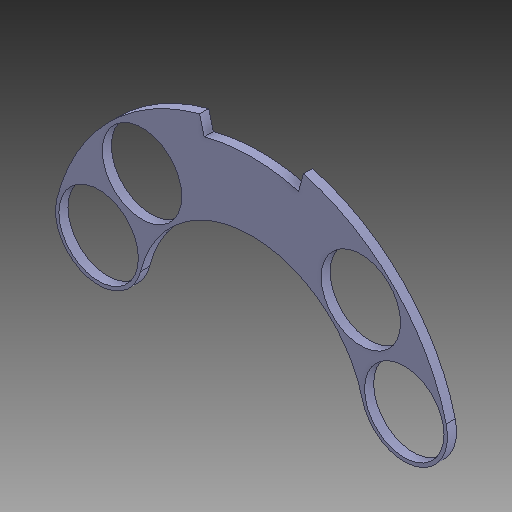
# Autodesk Inventor part: Диск_фиксатор
Saved by Autodesk Inventor 2022 (Build 260153000, 153)
## iProperties
Created: 2025-01-11
Part Number: Диск_фиксатор
Material: Типовые
Document SubType Name: Modeling
Designer: Ivan
Density: 1 g/cm^3
Appearance: Грифельно-синий
Mass: 52.9459 g
Surface Area: 260.986 cm^2
Volume: 52.9459 cm^3
Author: Ivan
Title: Диск_фиксатор
Autodesk Inventor part; units mm, degrees
ref_plane "YZ Plane" through (0, 0, 0) normal (1, 0, 0) x (0, 1, 0)
ref_plane "XZ Plane" through (0, 0, 0) normal (0, 1, 0) x (-1, 0, 0)
ref_plane "РабПлоскость2" through (0, 0, -38.7685) normal (0, 0, 1) x (-1, 0, 0)
sketch "Эскиз2" plane through (0, 0, -38.7685) normal (0, 0, 1) x (-1, 0, 0)
  line L0 (0, 0) -> (0, -166.5002) construction
  circle A0 centre (72.2445, -74.8113) radius 26 construction
  circle A1 centre (100.9108, -25.1599) radius 26 construction
  circle A2 centre (-72.2445, -74.8113) radius 26 construction
  circle A3 centre (-100.9108, -25.1599) radius 26 construction
  circle A4 centre (72.2445, -74.8113) radius 26.25
  circle A5 centre (100.9108, -25.1599) radius 26.25
  circle A6 centre (-72.2445, -74.8113) radius 26.25
  circle A7 centre (-100.9108, -25.1599) radius 26.25
  circle A8 centre (0, 0) radius 132.5 projected
  circle A9 centre (0, 0) radius 75.5
  circle A10 centre (100.9108, -25.1599) radius 28.5
  circle A11 centre (-100.9108, -25.1599) radius 28.5
  circle A12 centre (0, 0) radius 120.5
  line L1 (0, 0) -> (-34.2935, -127.9852)
  line L2 (0, 0) -> (34.2935, -127.9852)
  point P0 (-128.5642, -32.0547)
  point P1 (128.5642, -32.0547)
  point P2 (73.2573, -18.2651)
  point P3 (-73.2573, -18.2651)
  point P4 (-31.1877, -116.3941)
  point P5 (31.1877, -116.3941)
  dimension "d0" = 52.5
  dimension "d2" = 151
  dimension "d5" = 30
  dimension "d6" = 12
  constraints: 8 centre point, 8 coincident, 6 end point, 3 equal radius, 3 tangent, 2 point on circle, 1 vertical, 1 other
  measures "d0" diameter of A4
  measures "d2" diameter of A9
  measures "d5" angle of L2 L1
  measures "d6" radial gap between concentric circles of A12 A8
extrude "Выдавливание1" add sketch "Эскиз2" along normal blind 6 contours A4 A12 A10 A8 L2 | A4 A12 L2 A9 A10 | A12 A5 A10 | A10 A12 A5 | A12 L1 A9 L2 | L1 A8 A11 A12 A6 | A12 A6 A11 A9 L1 | A11 A12 A7 | A11 A12 A7
